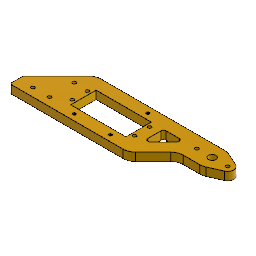
grt_shank_20190218 (Autodesk Fusion 360 archive; units mm, degrees)
design "grt_shank"
Autodesk Fusion 360 part; units mm, degrees
sketch "Skizze3" plane through (0, 0, 0) normal (0, 1, 0) x (1, 0, 0)
  line L0 (167.5736, -30) -> (33, -30)
  line L1 (31, -28) -> (31, -14.6863)
  line L2 (31.5858, -13.2721) -> (70.4645, 25.6066)
  line L3 (81.0711, 30) -> (230, 30)
  line L4 (199.3934, -4.3934) -> (178.1802, -25.6066)
  line L5 (210, 0) -> (230, 0)
  circle A0 centre (230, 15) radius 4.5
  circle A1 centre (211.5, 15) radius 2.1
  circle A2 centre (248.5, 15) radius 2.1
  circle A3 centre (248.5, 15) radius 7.5
  circle A4 centre (230, 15) radius 15
  line L6 (236.0811, 1.2879) -> (251.5405, 8.144)
  line L7 (251.3776, 21.926) -> (236.0828, 28.7113)
  arc A5 (167.5736, -30) -> (178.1802, -25.6066) centre (167.5736, -15) ccw
  arc A6 (210, 0) -> (199.3934, -4.3934) centre (210, -15) ccw
  arc A7 (81.0711, 30) -> (70.4645, 25.6066) centre (81.0711, 15) ccw
  arc A8 (31.5858, -13.2721) -> (31, -14.6863) centre (33, -14.6863) ccw
  arc A9 (31, -28) -> (33, -30) centre (33, -28) ccw
  line L8 (89.8088, -15.25) -> (156.3088, -15.25)
  line L9 (89.8088, 15.25) -> (89.8088, -15.25)
  line L10 (156.3088, -15.25) -> (156.3088, 15.25)
  line L11 (156.3088, 15.25) -> (89.8088, 15.25)
  circle A10 centre (160.5588, 9) radius 2.05
  circle A11 centre (85.5588, 9) radius 2.05
  circle A12 centre (85.5588, -9) radius 2.05
  circle A13 centre (160.5588, -9) radius 2.05
  line L12 (171.3088, 12) -> (171.3088, -4.0221)
  line L13 (176.4301, -6.1435) -> (192.4523, 9.8787)
  line L14 (190.331, 15) -> (174.3088, 15)
  arc A14 (174.3088, 15) -> (171.3088, 12) centre (174.3088, 12) ccw
  arc A15 (171.3088, -4.0221) -> (176.4301, -6.1435) centre (174.3088, -4.0221) ccw
  arc A16 (192.4523, 9.8787) -> (190.331, 15) centre (190.331, 12) ccw
  circle A17 centre (49, -20) radius 2.05
  circle A18 centre (69, 10) radius 2.05
  circle A19 centre (69, -20) radius 2.05
  dimension "d66" = 9
  dimension "d68" = 4.2
  dimension "d69" = 18.5
  dimension "d70" = 4.2
  dimension "d71" = 18.5
  dimension "d72" = 15
  dimension "d73" = 15
  dimension "d74" = 30
  dimension "d103" = 15
  dimension "d104" = 15
  dimension "d105" = 15
  dimension "d106" = 2
  dimension "d115" = 230
  dimension "d119" = 31
  dimension "d120" = 135
  dimension "d121" = 2
  dimension "d134" = 15.25
  dimension "d135" = 15.25
  dimension "d136" = 33.25
  dimension "d137" = 33.25
  dimension "d138" = 4.1
  dimension "d139" = 18
  dimension "d140" = 75
  dimension "d143" = 18.2
  dimension "d144" = 15.25
  dimension "d145" = 9
  dimension "d146" = 37.5
  dimension "d147" = 90
  dimension "d148" = 3
  dimension "d149" = 3
  dimension "d150" = 3
  dimension "d169" = 4.1
  dimension "d170" = 10
  dimension "d171" = 30
  dimension "d172" = 10
  dimension "d173" = 18
  dimension "d174" = 20
  dimension "d175" = 60
  dimension "d176" = 135
  dimension "d177" = 15
  dimension "d178" = 15
  dimension "d179" = 20
  dimension "d180" = 15
  measures "d66" diameter of A0
  measures "d68" diameter of A1
  measures "d70" diameter of A2
  measures "d73" diameter of A3
  measures "d74" diameter of A4
  measures "d103" radius of A5
  measures "d104" radius of A6
  measures "d105" radius of A7
  measures "d106" radius of A9
  measures "d115" distance of origin
  measures "d119" distance of origin L1
  measures "d120" angle of L1 L2
  measures "d121" radius of A8
  measures "d134" distance of origin L8
  measures "d135" distance of origin L11
  measures "d136" distance of origin L10
  measures "d137" distance of origin L9
  measures "d138" diameter of A13
  measures "d144" distance of origin L8
  measures "d145" distance of origin
  measures "d146" distance of origin
  measures "d147" distance of origin
  measures "d148" radius of A14
  measures "d149" radius of A15
  measures "d150" radius of A16
  measures "d169" diameter of A19
  measures "d170" distance of L2
  measures "d171" distance of origin
  measures "d173" distance of L1 origin
  measures "d175" distance of L0 L3
  measures "d176" angle of L0 L4
  measures "d177" distance of L4 L13
  measures "d178" distance of L3 L14
  measures "d180" distance of L10 L12
extrude "Extrusion16" add sketch "Skizze3" along normal blind 10
sketch "Skizze7" plane through (0, 10, 0) normal (0, 1, 0) x (-1, 0, 0)
  circle A0 centre (-248.5, -15) radius 2.1
  circle A1 centre (-85.5588, -9) radius 2.05
  line L0 (-89.8088, -15.25) -> (-156.3088, -15.25)
  line L1 (-156.3088, -15.25) -> (-156.3088, 15.25)
  line L2 (-156.3088, 15.25) -> (-89.8088, 15.25)
  line L3 (-89.8088, 15.25) -> (-89.8088, -15.25)
  circle A2 centre (-160.5588, 9) radius 2.05
  circle A3 centre (-85.5588, 9) radius 2.05
  circle A4 centre (-211.5, -15) radius 2.1
  circle A5 centre (-160.5588, -9) radius 2.05
  circle A6 centre (-230, -15) radius 4.5
  arc A7 (-192.4523, -9.8787) -> (-190.331, -15) centre (-190.331, -12) ccw
  line L4 (-192.4523, -9.8787) -> (-176.4301, 6.1435)
  arc A8 (-171.3088, 4.0221) -> (-176.4301, 6.1435) centre (-174.3088, 4.0221) ccw
  line L5 (-171.3088, 4.0221) -> (-171.3088, -12)
  arc A9 (-174.3088, -15) -> (-171.3088, -12) centre (-174.3088, -12) ccw
  line L6 (-174.3088, -15) -> (-190.331, -15)
  arc A10 (-31.5858, 13.2721) -> (-31, 14.6863) centre (-33, 14.6863) ccw
  line L7 (-31, 14.6863) -> (-31, 28)
  arc A11 (-31, 28) -> (-33, 30) centre (-33, 28) ccw
  line L8 (-33, 30) -> (-167.5736, 30)
  arc A12 (-167.5736, 30) -> (-178.1802, 25.6066) centre (-167.5736, 15) ccw
  line L9 (-178.1802, 25.6066) -> (-199.3934, 4.3934)
  arc A13 (-210, 0) -> (-199.3934, 4.3934) centre (-210, 15) ccw
  line L10 (-210, 0) -> (-230, 0)
  arc A14 (-230, 0) -> (-236.0811, -1.2879) centre (-230, -15) ccw
  line L11 (-236.0811, -1.2879) -> (-251.5405, -8.144)
  arc A15 (-251.5405, -8.144) -> (-251.3776, -21.926) centre (-248.5, -15) ccw
  line L12 (-251.3776, -21.926) -> (-236.0828, -28.7113)
  arc A16 (-236.0828, -28.7113) -> (-230, -30) centre (-230, -15) ccw
  line L13 (-230, -30) -> (-81.0711, -30)
  arc A17 (-81.0711, -30) -> (-70.4645, -25.6066) centre (-81.0711, -15) ccw
  line L14 (-70.4645, -25.6066) -> (-31.5858, 13.2721)
  line L15 (-143.8088, 21) -> (-145.8088, 21)
  line L16 (-146.3088, 21.5) -> (-146.3088, 23.5)
  line L17 (-145.8088, 24) -> (-143.8088, 24)
  line L18 (-143.3088, 23.5) -> (-143.3088, 21.5)
  arc A18 (-146.3088, 21.5) -> (-145.8088, 21) centre (-145.8088, 21.5) ccw
  arc A19 (-143.8088, 21) -> (-143.3088, 21.5) centre (-143.8088, 21.5) ccw
  arc A20 (-143.3088, 23.5) -> (-143.8088, 24) centre (-143.8088, 23.5) ccw
  arc A21 (-145.8088, 24) -> (-146.3088, 23.5) centre (-145.8088, 23.5) ccw
  line L19 (-102.3088, 24) -> (-100.3088, 24)
  arc A22 (-99.8088, 23.5) -> (-100.3088, 24) centre (-100.3088, 23.5) ccw
  arc A23 (-100.3088, 21) -> (-99.8088, 21.5) centre (-100.3088, 21.5) ccw
  line L20 (-100.3088, 21) -> (-102.3088, 21)
  arc A24 (-102.3088, 24) -> (-102.8088, 23.5) centre (-102.3088, 23.5) ccw
  line L21 (-99.8088, 23.5) -> (-99.8088, 21.5)
  arc A25 (-102.8088, 21.5) -> (-102.3088, 21) centre (-102.3088, 21.5) ccw
  line L22 (-102.8088, 21.5) -> (-102.8088, 23.5)
  line L23 (-145.8088, -21) -> (-143.8088, -21)
  arc A26 (-143.3088, -21.5) -> (-143.8088, -21) centre (-143.8088, -21.5) ccw
  arc A27 (-143.8088, -24) -> (-143.3088, -23.5) centre (-143.8088, -23.5) ccw
  line L24 (-143.8088, -24) -> (-145.8088, -24)
  arc A28 (-145.8088, -21) -> (-146.3088, -21.5) centre (-145.8088, -21.5) ccw
  line L25 (-143.3088, -21.5) -> (-143.3088, -23.5)
  arc A29 (-146.3088, -23.5) -> (-145.8088, -24) centre (-145.8088, -23.5) ccw
  line L26 (-146.3088, -23.5) -> (-146.3088, -21.5)
  circle A30 centre (-49, 20) radius 2.05
  circle A31 centre (-69, -10) radius 2.05
  circle A32 centre (-69, 20) radius 2.05
  dimension "d151" = 3
  dimension "d152" = 3
  dimension "d153" = 6
  dimension "d154" = 0.5
  dimension "d155" = 3
  dimension "d156" = 3
  dimension "d157" = 0.5
  dimension "d158" = 6
  dimension "d159" = 10
  dimension "d160" = 10
  dimension "d163" = 3
  dimension "d164" = 3
  dimension "d165" = 0.5
  dimension "d166" = 6
  dimension "d167" = 10
  measures "d154" radius of A18
  measures "d157" radius of A25
  measures "d158" distance of L8 L19
  measures "d159" distance of L3 L21
  measures "d160" distance of L1 L16
  measures "d165" radius of A29
  measures "d166" distance of L13 L24
  measures "d167" distance of L1 L26
extrude "Extrusion18" cut sketch "Skizze7" against normal blind 10 contours L15 L16 L17 L18 A18 A19 A20 A21 | L19 A22 A23 L20 A24 L21 A25 L22 | L23 A26 A27 L24 A28 L25 A29 L26
equation "d134 = 15 mm + tolerance"
equation "d135 = 15 mm + tolerance"
equation "d136 = 33 mm + tolerance"
equation "d137 = 33 mm + tolerance"
equation "d144 = 15 mm + tolerance"
equation "tolerance = 0.25 mm"
